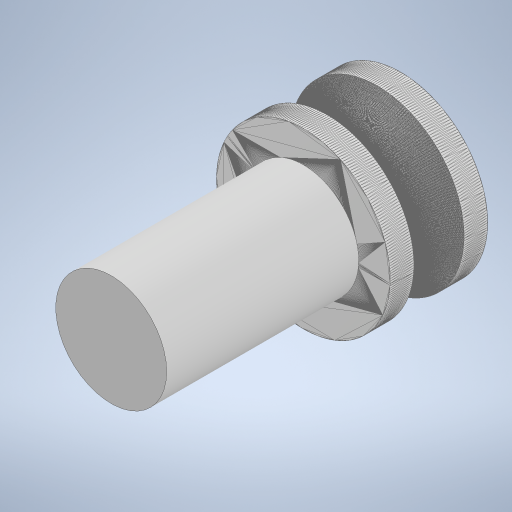
# Autodesk Inventor part: bearing-nairin
Saved by Autodesk Inventor 2024 (Build 280153000, 153)
## iProperties
Created: 2024-02-10
Part Number: bearing-nairin
Material: 一般
Document SubType Name: Modeling
Designer: mott1
Density: 1 g/cm^3
Appearance: 既定
Author: mott1
Autodesk Inventor part; units mm, degrees
ref_plane "YZ Plane" through (0, 0, 0) normal (1, 0, 0) x (0, 1, 0)
ref_plane "XZ Plane" through (0, 0, 0) normal (0, 1, 0) x (-1, 0, 0)
ref_plane "XY Plane" through (0, 0, 0) normal (0, 0, 1) x (1, 0, 0)
sketch "スケッチ1" plane through (-5.8121, -5.5336, 4.5) normal (0, 0, 1) x (1, 0, 0)
  circle A0 centre (5.8121, 5.5336) radius 5.1223
  constraints: 1 centre point, 1 coincident
extrude "押し出し1" add sketch "スケッチ1" along normal blind 17.75 and the other way blind 9
sketch "スケッチ2" plane through (0, 0, -4.5) normal (0, 0, -1) x (-1, 0, 0)
  circle A0 centre (0, 0) radius 2
  dimension "d4" = 4
  constraints: 1 centre point, 1 coincident
  measures "d4" diameter of A0
extrude "押し出し2" cut sketch "スケッチ2" against normal blind 2.5
